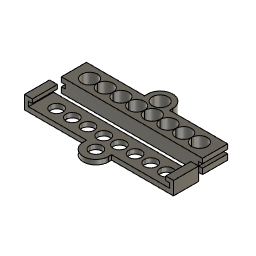
linear-holder (Autodesk Fusion 360 design; units mm, degrees)
Autodesk Fusion 360 part; units mm, degrees
sketch "Sketch1" plane through (0, 0, 0) normal (0, 0, 1) x (1, 0, 0)
  line L0 (-45, -10) -> (45, -10)
  line L1 (45, -10) -> (45, 10)
  line L2 (45, 10) -> (-45, 10)
  line L3 (-45, 10) -> (-45, -10)
  line L4 (-45, -10) -> (45, 10) construction
  line L5 (45, -10) -> (-45, 10) construction
  circle A0 centre (-5, 0) radius 5
  circle A1 centre (-15, 0) radius 5
  circle A2 centre (-25, 0) radius 5
  circle A3 centre (-35, 0) radius 5
  circle A4 centre (5, 0) radius 5
  circle A5 centre (15, 0) radius 5
  circle A6 centre (25, 0) radius 5
  circle A7 centre (35, 0) radius 5
  circle A8 centre (-5, 0) radius 4
  circle A9 centre (-15, 0) radius 4
  circle A10 centre (-25, 0) radius 4
  circle A11 centre (-35, 0) radius 4
  circle A12 centre (35, 0) radius 4
  circle A13 centre (25, 0) radius 4
  circle A14 centre (15, 0) radius 4
  circle A15 centre (5, 0) radius 4
  dimension "d1" = 90
  dimension "d2" = 20
  dimension "d3" = 10
  dimension "d6" = -30
  dimension "d7" = 0
  dimension "d10" = -30
  dimension "d11" = 0
  constraint horizontal L0
  constraint perpendicular L0 L1
  constraint parallel L0 L2
  constraint parallel L1 L3
  constraint coincident L4 origin
  constraint coincident L5 origin
  constraint concentric A0 A8
  measures "d1" distance of L1.end L2.end
  measures "d2" distance of L0.end L1.end
  measures "d3" diameter of A0
extrude "Extrude1" add sketch "Sketch1" against normal blind 7 contours L0 L1 L2 L3 makes body 1
extrude "Extrude2" add sketch "Sketch1" along normal blind 2 contours L0 L1 L2 L3 | A0 | A3 | A2 | A1 | A7 | A6 | A5 | A4 bodies 1
sketch "Sketch2" plane through (0, -10, 0) normal (0, -1, 0) x (1, 0, 0)
  line L0 (-45, 2) -> (-45, -7)
  line L1 (-45, -7) -> (45, -7)
  line L2 (45, -7) -> (45, 2)
  line L3 (45, 2) -> (-45, 2)
  line L4 (0, 2) -> (0, -7)
  line L5 (-45, -4) -> (-42.5, -4)
  line L6 (-42.5, -4) -> (-42.5, -1.5)
  line L7 (-42.5, -1.5) -> (-45, -1.5)
  line L8 (-45, -1.5) -> (-45, -4)
  line L9 (-45, -1.5) -> (-47.5, -1.5)
  line L10 (-47.5, -1.5) -> (-47.5, -7)
  line L11 (-47.5, -7) -> (-45, -7)
  line L12 (-45, -7) -> (-45, -1.5)
  line L13 (-47.5, -7) -> (0, -7)
  line L14 (0, -7) -> (0, -10)
  line L15 (0, -10) -> (-47.5, -10)
  line L16 (-47.5, -10) -> (-47.5, -7)
  line L17 (0, -10) -> (47.5, -10)
  line L18 (47.5, -10) -> (47.5, -7)
  line L19 (0, -7) -> (0, -10)
  line L20 (47.5, -7) -> (0, -7)
  line L21 (47.5, -1.5) -> (47.5, -7)
  line L22 (45, -7) -> (45, -1.5)
  line L23 (45, -4) -> (42.5, -4)
  line L24 (42.5, -4) -> (42.5, -1.5)
  line L25 (42.5, -1.5) -> (45, -1.5)
  line L26 (45, -1.5) -> (47.5, -1.5)
  dimension "d16" = 2.5
  dimension "d17" = 2.5
  dimension "d18" = 3
  dimension "d19" = 2.5
  dimension "d20" = 5.5
  constraint midpoint L3 L4.start
  constraint midpoint L1 L4.end
  constraint horizontal L5
  constraint vertical L6
  constraint horizontal L7
  constraint vertical L8
  constraint coincident L0 L5.start
  constraint horizontal L9
  constraint vertical L10
  constraint horizontal L11
  constraint vertical L12
  constraint horizontal L13
  constraint vertical L14
  constraint horizontal L15
  constraint vertical L16
  constraint symmetric L4 L5.start L23.start
  constraint symmetric L4 L5.end L23.end
  constraint symmetric L4 L6.end L24.end
  constraint symmetric L4 L7.end L22.end
  constraint symmetric L4 L9.end L21.start
  constraint symmetric L4 L10.end L18.end
  constraint symmetric L4 L0.end L1.end
  constraint symmetric L4 L13.end L14.start
  constraint symmetric L4 L14.end L15.start
  constraint symmetric L4 L15.end L17.end
  measures "d16" distance of L5.start L5.end
  measures "d17" distance of L5.start L7.end
  measures "d18" distance of L1 L5
  measures "d19" distance of L7.end L9.end
  measures "d20" distance of L7.end L0.end
sketch "Sketch3" plane through (0, 0, -7) normal (0, 0, -1) x (1, 0, 0)
  circle A0 centre (35, 0) radius 5
  arc A1 (20, 0) -> (30, 0) centre (25, 0) ccw
  arc A2 (10, 0) -> (20, 0) centre (15, 0) ccw
  arc A3 (0, 0) -> (10, 0) centre (5, 0) ccw
  arc A4 (-10, 0) -> (0, 0) centre (-5, 0) ccw
  arc A5 (-20, 0) -> (-10, 0) centre (-15, 0) ccw
  arc A6 (-30, 0) -> (-20, 0) centre (-25, 0) ccw
  circle A7 centre (-35, 0) radius 5
  arc A8 (-20, 0) -> (-30, 0) centre (-25, 0) ccw
  arc A9 (-10, 0) -> (-20, 0) centre (-15, 0) ccw
  arc A10 (0, 0) -> (-10, 0) centre (-5, 0) ccw
  arc A11 (10, 0) -> (0, 0) centre (5, 0) ccw
  arc A12 (20, 0) -> (10, 0) centre (15, 0) ccw
  arc A13 (30, 0) -> (20, 0) centre (25, 0) ccw
  line L0 (-45, 10) -> (-45, -10)
  line L1 (-45, -10) -> (45, -10)
  line L2 (45, -10) -> (45, 10)
  line L3 (45, 10) -> (-45, 10)
  circle A14 centre (-35, 0) radius 4
  circle A15 centre (-25, 0) radius 4
  circle A16 centre (-15, 0) radius 4
  circle A17 centre (-5, 0) radius 4
  circle A18 centre (5, 0) radius 4
  circle A19 centre (15, 0) radius 4
  circle A20 centre (25, 0) radius 4
  circle A21 centre (35, 0) radius 4
  dimension "d23" = 70
  dimension "d24" = 0
  dimension "d28" = 8
  constraint concentric A7 A14
  measures "d28" diameter of A21
extrude "Extrude3" cut sketch "Sketch2" against normal through all contours L0 L5 L6 L7 L8 L12 | L2 L22 L23 L24 L25 bodies 1
extrude "Extrude4" add sketch "Sketch2" against normal blind 20 separate body contours L0 L5 L6 L7 L8 L12 | L0 L8 L9 L10 L11 L12 L13 | L1 L11 L13 L14 L15 L16 L19 | L1 L14 L17 L18 L19 L20 | L2 L20 L21 L22 L26 | L2 L22 L23 L24 L25 makes body 2
extrude "Extrude5" cut sketch "Sketch3" along normal through all contours A14 | A15 | A16 | A17 | A18 | A19 | A20 | A21 bodies 2
sketch "Sketch4" plane through (0, 0, 2) normal (0, 0, 1) x (-1, 0, 0)
  circle A0 centre (-25, 0) radius 4
  circle A1 centre (35, 0) radius 4
  circle A2 centre (5, 0) radius 4
  circle A3 centre (-35, 0) radius 4
  circle A4 centre (25, 0) radius 4
  circle A5 centre (15, 0) radius 4
  circle A6 centre (-15, 0) radius 4
  circle A7 centre (-5, 0) radius 4
  line L0 (45, -10) -> (45, 10)
  line L1 (45, 10) -> (-45, 10)
  line L2 (-45, 10) -> (-45, -10)
  line L3 (-45, -10) -> (45, -10)
sketch "Sketch5" plane through (0, 0, 2) normal (0, 0, 1) x (1, 0, 0)
  circle A0 centre (0, -10) radius 5
  circle A1 centre (0, -10) radius 4
  line L0 (-8, -18) -> (8, -18)
  line L1 (8, -18) -> (8, -2)
  line L2 (8, -2) -> (-8, -2)
  line L3 (-8, -2) -> (-8, -18)
  line L4 (-8, -18) -> (8, -2) construction
  line L5 (8, -18) -> (-8, -2) construction
  line L6 (-8, -10) -> (8, -10)
  point P0 (0, -10)
  dimension "d30" = 8
  dimension "d31" = 16
  constraint concentric A0 A1
  constraint horizontal L0
  constraint perpendicular L0 L1
  constraint parallel L0 L2
  constraint parallel L1 L3
  constraint coincident L4 P0
  constraint coincident L5 P0
  constraint coincident P0 A0.centre
  constraint midpoint L3 L6.start
  constraint midpoint L1 L6.end
  measures "d30" diameter of A1
  measures "d31" distance of L0.end L1.end
sketch "Sketch6" plane through (0, -10, 0) normal (0, -1, 0) x (1, 0, 0)
  line L0 (45, -7) -> (-45, -7)
  line L1 (-45, -7) -> (-45, -4)
  line L2 (-45, -4) -> (-42.5, -4)
  line L3 (-42.5, -4) -> (-42.5, -1.5)
  line L4 (-42.5, -1.5) -> (-47.5, -1.5)
  line L5 (-47.5, -1.5) -> (-47.5, -10)
  line L6 (-47.5, -10) -> (47.5, -10)
  line L7 (47.5, -10) -> (47.5, -1.5)
  line L8 (47.5, -1.5) -> (42.5, -1.5)
  line L9 (42.5, -1.5) -> (42.5, -4)
  line L10 (42.5, -4) -> (45, -4)
  line L11 (45, -4) -> (45, -7)
  line L12 (-8, -10) -> (8, -10)
  line L13 (8, -10) -> (8, -7)
  line L14 (8, -7) -> (-8, -7)
  line L15 (-8, -7) -> (-8, -10)
  dimension "d32" = 16
  constraint horizontal L12
  constraint vertical L13
  constraint horizontal L14
  constraint vertical L15
  constraint coincident L6 L12.start
  measures "d32" distance of L12.start L12.end
extrude "Extrude6" add sketch "Sketch6" along normal blind 8 contours L0 L6 L12 L13 L14 L15 bodies 2
extrude "Extrude7" cut sketch "Sketch5" against normal through all contours A1 L6 | A1 L6 bodies 1 2
extrude "Extrude8" cut sketch "Sketch5" against normal blind 9 contours A0 A1 L6 | A0 A1 L6 bodies 1
extrude "Extrude9" add sketch "Sketch5" against normal blind 2 contours A0 A1 L6 | A0 A1 L6 bodies 1 2
extrude "Extrude10" add sketch "Sketch5" against normal blind 9 separate body contours A0 L0 L1 L3 L6 makes body 3
combine "Combine1" operation add target body 1 tool bodies 3
fillet "Fillet1" radius 8 2 edges at (8, -18, -2.5) (-8, -18, -2.5) on bodies 1
fillet "Fillet2" radius 8 2 edges at (8, -18, -8.5) (-8, -18, -8.5) on bodies 2
extrude "Extrude11" cut 2 faces at (-14.1667, 10, 0.8333) (-15, 10, -9) along direction (0, -1, 0) blind 2 on bodies 1 2 bodies 1 2
extrude "Extrude12" cut 4 faces at (19.5, -10, -2.1667) (33.5, -10, -9) (-19.5, -10, -2.1667) (-33.5, -10, -9) along direction (0, 1, 0) blind 2 on bodies 1 2 bodies 1 2
copy_body "Body->Comp1" bodies 1 removing the originals makes body 4 in component "Component"
copy_body "Body->Comp2" bodies 2 removing the originals makes body 5 in component "Component'"
move_body "Move1" bodies 4 to x (1, 0, 0) y (0, 1, 0) z (0, 0, 1) at (0, 28, -3) in component "Component"
move_body "Move2" bodies 4 to x (1, 0, 0) y (0, -1, 0) z (0, 0, -1) at (0, 45, -11) in component "Component"
move_body "Move3" bodies 4 to x (1, 0, 0) y (0, 1, 0) z (0, 0, 1) at (0, 1, 0) in component "Component"
move_body "Move4" bodies 4 to x (1, 0, 0) y (0, 1, 0) z (0, 0, 1) at (0, 3, 0) in component "Component"
component "Component" placed x (1, 0, 0) y (0, 1, 0) z (0, 0, 1) at (0, 0, 0)
component "Component'" placed x (1, 0, 0) y (0, 1, 0) z (0, 0, 1) at (0, 0, 0)
equation "d1 = ( 10 * 8 ) * 1 mm + ( 5 + 5 ) * 1 mm"
equation "d2 = 10 mm + 10 mm"
